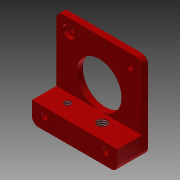
# Autodesk Inventor part: extruder_base
Saved by Autodesk Inventor 2013 (Build 170138000, 138)
## iProperties
Created: 2015-02-21
Part Number: extruder_base
Material: 一般
Document SubType Name: Modeling
Designer: Noa Izumi
Density: 1 g/cm^3
Author: Noa Izumi
Autodesk Inventor part; units mm, degrees
ref_plane "YZ Plane" through (0, 0, 0) normal (1, 0, 0) x (0, 1, 0)
ref_plane "XZ Plane" through (0, 0, 0) normal (0, 1, 0) x (-1, 0, 0)
ref_plane "XY Plane" through (0, 0, 0) normal (0, 0, 1) x (1, 0, 0)
sketch "草圖1" plane through (0, 0, 0) normal (0, 1, 0) x (-1, 0, 0)
  line L0 (0, 0) -> (42, 0)
  line L1 (42, 0) -> (42, 42)
  line L2 (42, 42) -> (0, 42)
  line L3 (0, 42) -> (0, 0)
  dimension "d0" = 42
  dimension "d1" = 42
  constraints: 8 end point, 2 parallel, 1 horizontal, 1 perpendicular
  measures "d0" distance of L0.start L0.end
  measures "d1" distance of L2.end L0.start
extrude "擠出1" add sketch "草圖1" along normal blind 3
sketch "草圖2" plane through (0, 0, 0) normal (0, -1, 0) x (1, 0, 0)
  line L0 (0, 0) -> (-42, 0) projected
  line L1 (0, 42) -> (0, 0) projected
  line L2 (-42, 0) -> (0, 0)
  line L3 (0, 0) -> (0, 10)
  line L4 (0, 10) -> (-42, 10)
  line L5 (-42, 10) -> (-42, 0)
  dimension "d4" = 10
  constraints: 8 end point, 2 parallel, 1 horizontal, 1 perpendicular, 1 point on line
  measures "d4" distance of L2.end L3.end
extrude "擠出2" add sketch "草圖2" along normal blind 12
sketch "草圖3" plane through (0, 3, 0) normal (0, 1, 0) x (1, 0, 0)
  point P0 (-21, -21)
hole "孔1" at (-21, 3, 21) direction (0, -1, 0) diameter 22 end through all
sketch "草圖4" plane through (0, 3, 0) normal (0, 1, 0) x (1, 0, 0)
  circle A0 centre (-21, -21) radius 11 projected
  point P0 (-36, -6)
  point P1 (-36, -36)
  point P2 (-6, -6)
  point P3 (-6, -36)
  dimension "d15" = 15
  dimension "d16" = 15
  dimension "d17" = 15
  dimension "d18" = 15
  measures "d15" horizontal distance of A0.centre point (-36, -6)
  measures "d16" horizontal distance of A0.centre point (-36, -6)
  measures "d17" horizontal distance of A0.centre point (-36, -36)
  measures "d18" horizontal distance of point (-6, -6) A0.centre
hole "孔2" at (-36, 3, 6) at (-36, 3, 36) at (-6, 3, 6) at (-6, 3, 36) direction (0, -1, 0) diameter 3 end through all
fillet "圓角1" radius 3 4 edges at (0, 1.5, 42) (0, -4.5, 0) (-42, 1.5, 42) (-42, -4.5, 0)
sketch "草圖5" plane through (0, 0, 0) normal (0, -1, 0) x (1, 0, 0)
  circle A0 centre (-36, 36) radius 1.5 projected
  point P0 (0, 0)
  constraints: 1 coincident
hole "孔3" at (-36, 0, 36) direction (0, 1, 0) diameter 6 depth 2
sketch "草圖6" plane through (-3, 3, 0) normal (0, 0, -1) x (-1, 0, 0)
  line L0 (0, 0) -> (36, 0) projected
  line L1 (-3, 0) -> (-3, -15) projected
  point P0 (-3, -3)
  point P1 (12, -7.5)
  dimension "d35" = 7.5
  dimension "d36" = 15
  measures "d35" distance from line of point (12, -7.5) L0
  measures "d36" distance from line of point (12, -7.5) L1
hole "孔4" at (-15, -4.5, 0) direction (0, 0, 1) diameter 4.917 end through all thread size "M6x1" class "6H" standard "ANSI Metric M Profile"
sketch "草圖7" plane through (-3, 3, 0) normal (0, 0, -1) x (-1, 0, 0)
  line L0 (39, -15) -> (39, 0) projected
  point P0 (-3, -3)
  point P1 (29, -7.5)
  dimension "d44" = 10
  measures "d44" distance from line of point (29, -7.5) L0
hole "孔5" at (-32, -4.5, 0) direction (0, 0, 1) diameter 3.242 end through all counterbore diameter 7.5 counterbore depth 2 thread size "M4x0.7" class "6H" standard "ANSI Metric M Profile"
